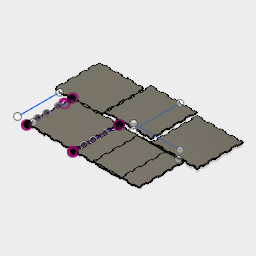
hezi2 v0 (Autodesk Fusion 360 design; units mm, degrees)
Autodesk Fusion 360 part; units mm, degrees
sketch "草图1" plane through (0, 0, 0) normal (0, 1, 0) x (1, 0, 0)
  line L0 (-50, 0) -> (30, 0)
  line L1 (30, 0) -> (30, -80)
  line L2 (30, -80) -> (-50, -80)
  line L3 (-50, -80) -> (-50, 0)
  line L4 (30, -10) -> (28, -10)
  line L5 (28, -10) -> (30, -10)
  line L6 (30, -10) -> (30, -20)
  line L7 (30, -20) -> (28, -20)
  line L8 (28, -20) -> (28, -10)
  line L9 (28, -30.1419) -> (30, -30.1419)
  line L10 (30, -30.1419) -> (30, -40)
  line L11 (30, -40) -> (28, -40)
  line L12 (28, -40) -> (28, -30.1419)
  line L13 (28, -49.9122) -> (30, -49.9122)
  line L14 (30, -49.9122) -> (30, -60)
  line L15 (30, -60) -> (28, -60)
  line L16 (28, -60) -> (28, -49.9122)
  line L17 (28, -70.124) -> (30, -70.124)
  line L18 (30, -70.124) -> (30, -80)
  line L19 (30, -80) -> (28, -80)
  line L20 (-50, -10) -> (-48, -10)
  line L21 (-48, -10) -> (-48, -19.9095)
  line L22 (-48, -19.9095) -> (-50, -19.9095)
  line L23 (-50, -19.9095) -> (-50, -10)
  line L24 (-48, -30.0089) -> (-50, -30.0089)
  line L25 (-50, -30.0089) -> (-50, -40)
  line L26 (-50, -40) -> (-48, -40)
  line L27 (-48, -40) -> (-48, -30.0089)
  line L28 (-48, -50.2335) -> (-50, -50.2335)
  line L29 (-50, -50.2335) -> (-50, -60)
  line L30 (-50, -60) -> (-48, -60)
  line L31 (-48, -60) -> (-48, -50.2335)
  line L32 (-50, -70.0828) -> (-50, -80)
  line L33 (-50, -80) -> (-48, -80)
  line L34 (-48, -70.0522) -> (-50, -70.0522)
  line L35 (-50, -70.0522) -> (-50, -75.0522)
  line L36 (-50, -75.0522) -> (-48, -75.0522)
  line L37 (-48, -75.0522) -> (-48, -70.0522)
  line L38 (28, -70.124) -> (30, -70.124)
  line L39 (30, -70.124) -> (30, -75.062)
  line L40 (30, -75.062) -> (28, -75.062)
  line L41 (28, -75.062) -> (28, -70.124)
  line L42 (-30, -80) -> (-19.728, -80)
  line L43 (-19.728, -80) -> (-19.728, -78)
  line L44 (-19.728, -78) -> (-30, -78)
  line L45 (-30, -78) -> (-30, -80)
  line L46 (-9.7551, -78) -> (0, -78)
  line L47 (0, -78) -> (0, -80)
  line L48 (0, -80) -> (-9.7551, -80)
  line L49 (-9.7551, -80) -> (-9.7551, -78)
  line L50 (-40.3031, -78) -> (-45.3133, -78)
  line L51 (-45.3133, -78) -> (-45.3133, -80)
  line L52 (-45.3133, -80) -> (-40.3031, -80)
  line L53 (-40.3031, -80) -> (-40.3031, -78)
  line L54 (-45.3133, 0) -> (-40.3031, 0)
  line L55 (-40.3031, 0) -> (-40.3031, -2)
  line L56 (-40.3031, -2) -> (-45.3133, -2)
  line L57 (-45.3133, -2) -> (-45.3133, 0)
  line L58 (-29.7585, -2) -> (-20, -2)
  line L59 (-20, -2) -> (-20, 0)
  line L60 (-20, 0) -> (-29.7585, 0)
  line L61 (-29.7585, 0) -> (-29.7585, -2)
  line L62 (-10, -2) -> (0, -2)
  line L63 (0, -2) -> (0, 0)
  line L64 (0, 0) -> (-10, 0)
  line L65 (-10, 0) -> (-10, -2)
  line L66 (10.2052, -2) -> (20, -2)
  line L67 (20, -2) -> (20, 0)
  line L68 (20, 0) -> (10.2052, 0)
  line L69 (10.2052, 0) -> (10.2052, -2)
  line L70 (10.3405, -78) -> (20, -78)
  line L71 (20, -78) -> (20, -80)
  line L72 (20, -80) -> (10.3405, -80)
  line L73 (10.3405, -80) -> (10.3405, -78)
  dimension "d1" = 80
  dimension "d2" = 80
  dimension "d3" = 2
  dimension "d4" = 2
  dimension "d5" = 5
  dimension "d6" = 2
  dimension "d7" = 2
  dimension "d8" = 2
  measures "d1" distance of L0.start L2.end
  measures "d2" distance of L0.start L0.end
  measures "d3" distance of L4.start L4.end
  measures "d4" distance of L20.start L20.end
  measures "d5" distance of L34.start L36.end
  measures "d6" distance of L17.start L17.end
  measures "d7" distance of L42.start L44.end
  measures "d8" distance of L54.start L56.end
extrude "拉伸1" add sketch "草图1" along normal blind 2 contours L0 L1 L2 L3 L4 L5 L7 L8 L9 L11 L12 L13 L15 L16 L17 L18 L19 L20 L21 L22 L24 L26 L27 L28 L30 L31 L32 L33 L34 L36 L37 L38 L40 L41 L43 L44 L45 L46 L47 L49 L50 L51 L53 L55 L56 L57 L58 L59 L61 L62 L63 L65 L66 L67 L69 L70 L71 L73 makes body 1
box "长方体基本要素1" add length 80 width 80 height 2 placed x (0, 0, 1) y (1, 0, 0) z (0, 1, 0) at (50, 0, 0) separate body makes body 2
sketch "草图3" plane through (0, 2, 0) normal (0, 1, 0) x (-1, 0, 0)
  line L0 (-50, 80) -> (-130, 80)
  line L1 (-130, 80) -> (-130, 0)
  line L2 (-130, 0) -> (-50, 0)
  line L3 (-50, 0) -> (-50, 80)
  line L4 (-50, 0) -> (-52, 0)
  line L5 (-52, 0) -> (-52, 9.9337)
  line L6 (-52, 9.9337) -> (-50, 9.9337)
  line L7 (-50, 9.9337) -> (-50, 0)
  line L8 (-52, 20.0066) -> (-50, 20.0066)
  line L9 (-50, 20.0066) -> (-50, 30)
  line L10 (-50, 30) -> (-52, 30)
  line L11 (-52, 30) -> (-52, 20.0066)
  line L12 (-52, 39.9379) -> (-50, 39.9379)
  line L13 (-50, 39.9379) -> (-50, 50)
  line L14 (-50, 50) -> (-52, 50)
  line L15 (-52, 50) -> (-52, 39.9379)
  line L16 (-52, 59.8692) -> (-50, 59.8692)
  line L17 (-50, 59.8692) -> (-50, 70)
  line L18 (-50, 70) -> (-52, 70)
  line L19 (-52, 70) -> (-52, 59.8692)
  line L20 (-52, 75.0856) -> (-50, 75.0856)
  line L21 (-50, 75.0856) -> (-50, 80)
  line L22 (-50, 80) -> (-52, 80)
  line L23 (-52, 80) -> (-52, 75.0856)
  line L24 (-130, 0) -> (-128, 0)
  line L25 (-128, 0) -> (-128, 9.9337)
  line L26 (-128, 9.9337) -> (-130, 9.9337)
  line L27 (-130, 9.9337) -> (-130, 0)
  line L28 (-128, 20.2209) -> (-130, 20.2209)
  line L29 (-130, 20.2209) -> (-130, 30)
  line L30 (-130, 30) -> (-128, 30)
  line L31 (-128, 30) -> (-128, 20.2209)
  line L32 (-128, 39.9379) -> (-130, 39.9379)
  line L33 (-130, 39.9379) -> (-130, 50)
  line L34 (-130, 50) -> (-128, 50)
  line L35 (-128, 50) -> (-128, 39.9379)
  line L36 (-128, 59.8692) -> (-130, 59.8692)
  line L37 (-130, 59.8692) -> (-130, 70)
  line L38 (-130, 70) -> (-128, 70)
  line L39 (-128, 70) -> (-128, 59.8692)
  line L40 (-128, 75.0856) -> (-130, 75.0856)
  line L41 (-130, 75.0856) -> (-130, 80)
  line L42 (-130, 80) -> (-128, 80)
  line L43 (-128, 80) -> (-128, 75.0856)
  line L44 (-55, 0) -> (-64.9634, 0)
  line L45 (-64.9634, 0) -> (-64.9634, 2)
  line L46 (-64.9634, 2) -> (-55, 2)
  line L47 (-55, 2) -> (-55, 0)
  line L48 (-75.0362, 2) -> (-85, 2)
  line L49 (-85, 2) -> (-85, 0)
  line L50 (-85, 0) -> (-75.0362, 0)
  line L51 (-75.0362, 0) -> (-75.0362, 2)
  line L52 (-94.9675, 2) -> (-105, 2)
  line L53 (-105, 2) -> (-105, 0)
  line L54 (-105, 0) -> (-94.9675, 0)
  line L55 (-94.9675, 0) -> (-94.9675, 2)
  line L56 (-109.9696, 2) -> (-120, 2)
  line L57 (-120, 2) -> (-120, 0)
  line L58 (-120, 0) -> (-109.9696, 0)
  line L59 (-109.9696, 0) -> (-109.9696, 2)
  line L60 (-55, 80) -> (-64.9634, 80)
  line L61 (-64.9634, 80) -> (-64.9634, 78)
  line L62 (-64.9634, 78) -> (-55, 78)
  line L63 (-55, 78) -> (-55, 80)
  line L64 (-75.2505, 78) -> (-85, 78)
  line L65 (-85, 78) -> (-85, 80)
  line L66 (-85, 80) -> (-75.2505, 80)
  line L67 (-75.2505, 80) -> (-75.2505, 78)
  line L68 (-94.9675, 78) -> (-105, 78)
  line L69 (-105, 78) -> (-105, 80)
  line L70 (-105, 80) -> (-94.9675, 80)
  line L71 (-94.9675, 80) -> (-94.9675, 78)
  line L72 (-109.9696, 78) -> (-120, 78)
  line L73 (-120, 78) -> (-120, 80)
  line L74 (-120, 80) -> (-109.9696, 80)
  line L75 (-109.9696, 80) -> (-109.9696, 78)
  dimension "d16" = 2
  measures "d16" distance of L2.end L4.end
extrude "拉伸2" add sketch "草图3" along normal blind 2 contours L0 L1 L2 L3 L5 L6 L8 L10 L11 L12 L14 L15 L16 L18 L19 L20 L23 L25 L26 L28 L30 L31 L32 L34 L35 L36 L38 L39 L40 L43 L45 L46 L47 L48 L49 L51 L52 L53 L55 L56 L57 L59 L61 L62 L63 L64 L65 L67 L68 L69 L71 L72 L73 L75 bodies 2
sketch "草图4" plane through (0, 0, 0) normal (0, 0, -1) x (-1, 0, 0)
  line L0 (-130, 2) -> (-130, 0)
  line L1 (-130, 0) -> (-50, 0)
  line L2 (-50, 0) -> (-50, 2)
  line L3 (-50, 2) -> (-52, 2)
  line L4 (-52, 2) -> (-52, 4)
  line L5 (-52, 4) -> (-55, 4)
  line L6 (-55, 4) -> (-55, 2)
  line L7 (-55, 2) -> (-64.9634, 2)
  line L8 (-64.9634, 2) -> (-64.9634, 4)
  line L9 (-64.9634, 4) -> (-75.0362, 4)
  line L10 (-75.0362, 4) -> (-75.0362, 2)
  line L11 (-75.0362, 2) -> (-85, 2)
  line L12 (-85, 2) -> (-85, 4)
  line L13 (-85, 4) -> (-94.9675, 4)
  line L14 (-94.9675, 4) -> (-94.9675, 2)
  line L15 (-94.9675, 2) -> (-105, 2)
  line L16 (-105, 2) -> (-105, 4)
  line L17 (-105, 4) -> (-109.9696, 4)
  line L18 (-109.9696, 4) -> (-109.9696, 2)
  line L19 (-109.9696, 2) -> (-120, 2)
  line L20 (-120, 2) -> (-120, 4)
  line L21 (-120, 4) -> (-128, 4)
  line L22 (-128, 4) -> (-128, 2)
  line L23 (-128, 2) -> (-130, 2)
  line L24 (-130, 2) -> (-50, 2)
  line L25 (-50, 2) -> (-50, 0)
  line L26 (-50, 0) -> (-130, 0)
  line L27 (-130, 0) -> (-130, 2)
extrude "拉伸3" cut sketch "草图4" against normal blind 80 contours L0 L1 L2 L3 L7 L11 L15 L19 L23 L24 L25 L26 L27 bodies 2
move_body "移动1" bodies 2 to x (1, 0, 0) y (0, 1, 0) z (0, 0, 1) at (0, -2, 0)
sketch "草图5" plane through (0, 2, 0) normal (0, 1, 0) x (-1, 0, 0)
  line L0 (9.7551, 80) -> (9.7551, 78)
  line L1 (9.7551, 78) -> (0, 78)
  line L2 (0, 78) -> (0, 80)
  line L3 (0, 80) -> (-10.3405, 80)
  line L4 (-10.3405, 80) -> (-10.3405, 78)
  line L5 (-10.3405, 78) -> (-20, 78)
  line L6 (-20, 78) -> (-20, 80)
  line L7 (-20, 80) -> (-30, 80)
  line L8 (-30, 80) -> (-30, 75.062)
  line L9 (-30, 75.062) -> (-28, 75.062)
  line L10 (-28, 75.062) -> (-28, 70.124)
  line L11 (-28, 70.124) -> (-30, 70.124)
  line L12 (-30, 70.124) -> (-30, 60)
  line L13 (-30, 60) -> (-28, 60)
  line L14 (-28, 60) -> (-28, 49.9122)
  line L15 (-28, 49.9122) -> (-30, 49.9122)
  line L16 (-30, 49.9122) -> (-30, 40)
  line L17 (-30, 40) -> (-28, 40)
  line L18 (-28, 40) -> (-28, 30.1419)
  line L19 (-28, 30.1419) -> (-30, 30.1419)
  line L20 (-30, 30.1419) -> (-30, 20)
  line L21 (-30, 20) -> (-28, 20)
  line L22 (-28, 20) -> (-28, 10)
  line L23 (-28, 10) -> (-30, 10)
  line L24 (-30, 10) -> (-30, 0)
  line L25 (-30, 0) -> (-20, 0)
  line L26 (-20, 0) -> (-20, 2)
  line L27 (-20, 2) -> (-10.2052, 2)
  line L28 (-10.2052, 2) -> (-10.2052, 0)
  line L29 (-10.2052, 0) -> (0, 0)
  line L30 (0, 0) -> (0, 2)
  line L31 (0, 2) -> (10, 2)
  line L32 (10, 2) -> (10, 0)
  line L33 (10, 0) -> (20, 0)
  line L34 (20, 0) -> (20, 2)
  line L35 (20, 2) -> (29.7585, 2)
  line L36 (29.7585, 2) -> (29.7585, 0)
  line L37 (29.7585, 0) -> (40.3031, 0)
  line L38 (40.3031, 0) -> (40.3031, 2)
  line L39 (40.3031, 2) -> (45.3133, 2)
  line L40 (45.3133, 2) -> (45.3133, 0)
  line L41 (45.3133, 0) -> (50, 0)
  line L42 (50, 0) -> (50, 10)
  line L43 (50, 10) -> (48, 10)
  line L44 (48, 10) -> (48, 19.9095)
  line L45 (48, 19.9095) -> (50, 19.9095)
  line L46 (50, 19.9095) -> (50, 30.0089)
  line L47 (50, 30.0089) -> (48, 30.0089)
  line L48 (48, 30.0089) -> (48, 40)
  line L49 (48, 40) -> (50, 40)
  line L50 (50, 40) -> (50, 50.2335)
  line L51 (50, 50.2335) -> (48, 50.2335)
  line L52 (48, 50.2335) -> (48, 60)
  line L53 (48, 60) -> (50, 60)
  line L54 (50, 60) -> (50, 70.0522)
  line L55 (50, 70.0522) -> (48, 70.0522)
  line L56 (48, 70.0522) -> (48, 75.0522)
  line L57 (48, 75.0522) -> (50, 75.0522)
  line L58 (50, 75.0522) -> (50, 80)
  line L59 (50, 80) -> (45.3133, 80)
  line L60 (45.3133, 80) -> (45.3133, 78)
  line L61 (45.3133, 78) -> (40.3031, 78)
  line L62 (40.3031, 78) -> (40.3031, 80)
  line L63 (40.3031, 80) -> (30, 80)
  line L64 (30, 80) -> (30, 78)
  line L65 (30, 78) -> (19.728, 78)
  line L66 (19.728, 78) -> (19.728, 80)
  line L67 (19.728, 80) -> (9.7551, 80)
  line L68 (50, 85) -> (-30, 85)
  line L69 (-30, 85) -> (-30, 165)
  line L70 (-30, 165) -> (50, 165)
  line L71 (50, 165) -> (50, 85)
  line L72 (50, 85) -> (45.3133, 85)
  line L73 (45.3133, 85) -> (45.3133, 87)
  line L74 (45.3133, 87) -> (50, 87)
  line L75 (50, 87) -> (50, 85)
  line L76 (40.0206, 87) -> (30.0852, 87)
  line L77 (30.0852, 87) -> (30.0852, 85)
  line L78 (30.0852, 85) -> (40.0206, 85)
  line L79 (40.0206, 85) -> (40.0206, 87)
  line L80 (19.9188, 87) -> (10, 87)
  line L81 (10, 87) -> (10, 85)
  line L82 (10, 85) -> (19.9188, 85)
  line L83 (19.9188, 85) -> (19.9188, 87)
  line L84 (0.048, 87) -> (-10.5806, 87)
  line L85 (-10.5806, 87) -> (-10.5806, 85)
  line L86 (-10.5806, 85) -> (0.048, 85)
  line L87 (0.048, 85) -> (0.048, 87)
  line L88 (-20.2849, 87) -> (-30, 87)
  line L89 (-30, 87) -> (-30, 85)
  line L90 (-30, 85) -> (-20.2849, 85)
  line L91 (-20.2849, 85) -> (-20.2849, 87)
  line L92 (45.3133, 165) -> (50, 165)
  line L93 (50, 165) -> (50, 163)
  line L94 (50, 163) -> (45.3133, 163)
  line L95 (45.3133, 163) -> (45.3133, 165)
  line L96 (40.0206, 163) -> (29.8542, 163)
  line L97 (29.8542, 163) -> (29.8542, 165)
  line L98 (29.8542, 165) -> (40.0206, 165)
  line L99 (40.0206, 165) -> (40.0206, 163)
  line L100 (19.9188, 163) -> (10, 163)
  line L101 (10, 163) -> (10, 165)
  line L102 (10, 165) -> (19.9188, 165)
  line L103 (19.9188, 165) -> (19.9188, 163)
  line L104 (-0.1831, 163) -> (-10.1185, 163)
  line L105 (-10.1185, 163) -> (-10.1185, 165)
  line L106 (-10.1185, 165) -> (-0.1831, 165)
  line L107 (-0.1831, 165) -> (-0.1831, 163)
  line L108 (-20.0539, 163) -> (-30, 163)
  line L109 (-30, 163) -> (-30, 165)
  line L110 (-30, 165) -> (-20.0539, 165)
  line L111 (-20.0539, 165) -> (-20.0539, 163)
  dimension "d21" = 80
  dimension "d22" = 80
  dimension "d23" = 2
  dimension "d24" = 2
  measures "d21" distance of L68.start L70.end
  measures "d22" distance of L68.start L68.end
  measures "d23" distance of L68.start L74.end
  measures "d24" distance of L92.start L94.end
move_body "移动2" bodies 2 to x (1, 0, 0) y (0, 1, 0) z (0, 0, 1) at (0, 0, 85)
sketch "草图6" plane through (0, 0, 0) normal (0, 1, 0) x (1, 0, 0)
  line L0 (30, -85) -> (30, -165)
  line L1 (30, -85) -> (132.5104, -85)
  point P0 (30, -85)
move_face "MoveFace1" to x (0, 0, 1) y (0, 1, 0) z (-1, 0, 0) at (174.9428, 0, 36.9961) 1 faces at (91.6558, 2, 137.6253) on bodies 2
move_body "移动3" bodies 2 to x (0, 0, 1) y (0, 1, 0) z (-1, 0, 0) at (197.9117, 0, 33.4081)
move_body "移动4" bodies 2 to x (1, 0, 0) y (0, 1, 0) z (0, 0, 1) at (0, 0, 2)
sketch "草图7" plane through (0, 0, 0) normal (0, 1, 0) x (1, 0, 0)
  line L0 (30, -87) -> (28, -87)
  line L1 (28, -87) -> (28, -90.3428)
  line L2 (28, -90.3428) -> (30, -90.3428)
  line L3 (30, -90.3428) -> (30, -87)
  line L4 (28, -100.0471) -> (30, -100.0471)
  line L5 (30, -100.0471) -> (30, -110)
  line L6 (30, -110) -> (28, -110)
  line L7 (28, -110) -> (28, -100.0471)
  line L8 (30, -85) -> (30, -165)
  line L9 (28, -120.38) -> (30, -120.38)
  line L10 (30, -120.38) -> (30, -130)
  line L11 (30, -130) -> (28, -130)
  line L12 (28, -130) -> (28, -120.38)
  line L13 (28, -140.2508) -> (30, -140.2508)
  line L14 (30, -140.2508) -> (30, -145.334)
  line L15 (30, -145.334) -> (28, -145.334)
  line L16 (28, -145.334) -> (28, -140.2508)
  line L17 (28, -155.5004) -> (30, -155.5004)
  line L18 (30, -155.5004) -> (30, -163)
  line L19 (30, -163) -> (28, -163)
  line L20 (28, -163) -> (28, -155.5004)
  line L21 (-50, -87) -> (-48, -87)
  line L22 (-48, -87) -> (-48, -90.3428)
  line L23 (-48, -90.3428) -> (-50, -90.3428)
  line L24 (-50, -90.3428) -> (-50, -87)
  line L25 (-48, -100.2781) -> (-50, -100.2781)
  line L26 (-50, -100.2781) -> (-50, -110)
  line L27 (-50, -110) -> (-48, -110)
  line L28 (-48, -110) -> (-48, -100.2781)
  line L29 (-50, -165) -> (-50, -85)
  line L30 (-48, -119.9179) -> (-50, -119.9179)
  line L31 (-50, -119.9179) -> (-50, -130)
  line L32 (-50, -130) -> (-48, -130)
  line L33 (-48, -130) -> (-48, -119.9179)
  line L34 (-48, -140.2508) -> (-50, -140.2508)
  line L35 (-50, -140.2508) -> (-50, -145.334)
  line L36 (-50, -145.334) -> (-48, -145.334)
  line L37 (-48, -145.334) -> (-48, -140.2508)
  line L38 (-50, -163) -> (-48, -163)
  line L39 (-48, -155.5004) -> (-50, -155.5004)
  line L40 (-50, -155.5004) -> (-50, -163)
  line L41 (-50, -155.5004) -> (-48, -155.5004)
  line L42 (-48, -155.5004) -> (-48, -163)
  line L43 (-48, -163) -> (-50, -163)
  line L44 (-50, -163) -> (-50, -155.5004)
  point P0 (30, -87)
  point P1 (30, -163)
  point P2 (-50, -87)
  point P3 (-50, -163)
  dimension "d25" = 2
  dimension "d26" = 2
  measures "d25" distance of P0 L0.end
  measures "d26" distance of P3 L38.end
extrude "拉伸4" add sketch "草图5" along normal blind 2 separate body contours L68 L69 L70 L71 L73 L74 L76 L77 L79 L80 L81 L83 L84 L85 L87 L88 L91 L94 L95 L96 L97 L99 L100 L101 L103 L104 L105 L107 L108 L111 makes body 3
sketch "草图8" plane through (0, 4, 0) normal (0, 1, 0) x (-1, 0, 0)
  line L0 (-0.1831, 165) -> (-0.1831, 163)
  line L1 (-0.1831, 163) -> (-10.1185, 163)
  line L2 (-10.1185, 163) -> (-10.1185, 165)
  line L3 (-10.1185, 165) -> (-20.0539, 165)
  line L4 (-20.0539, 165) -> (-20.0539, 163)
  line L5 (-20.0539, 163) -> (-30, 163)
  line L6 (-30, 163) -> (-30, 87)
  line L7 (-30, 87) -> (-20.2849, 87)
  line L8 (-20.2849, 87) -> (-20.2849, 85)
  line L9 (-20.2849, 85) -> (-10.5806, 85)
  line L10 (-10.5806, 85) -> (-10.5806, 87)
  line L11 (-10.5806, 87) -> (0.048, 87)
  line L12 (0.048, 87) -> (0.048, 85)
  line L13 (0.048, 85) -> (10, 85)
  line L14 (10, 85) -> (10, 87)
  line L15 (10, 87) -> (19.9188, 87)
  line L16 (19.9188, 87) -> (19.9188, 85)
  line L17 (19.9188, 85) -> (30.0852, 85)
  line L18 (30.0852, 85) -> (30.0852, 87)
  line L19 (30.0852, 87) -> (40.0206, 87)
  line L20 (40.0206, 87) -> (40.0206, 85)
  line L21 (40.0206, 85) -> (45.3133, 85)
  line L22 (45.3133, 85) -> (45.3133, 87)
  line L23 (45.3133, 87) -> (50, 87)
  line L24 (50, 87) -> (50, 163)
  line L25 (50, 163) -> (45.3133, 163)
  line L26 (45.3133, 163) -> (45.3133, 165)
  line L27 (45.3133, 165) -> (40.0206, 165)
  line L28 (40.0206, 165) -> (40.0206, 163)
  line L29 (40.0206, 163) -> (29.8542, 163)
  line L30 (29.8542, 163) -> (29.8542, 165)
  line L31 (29.8542, 165) -> (19.9188, 165)
  line L32 (19.9188, 165) -> (19.9188, 163)
  line L33 (19.9188, 163) -> (10, 163)
  line L34 (10, 163) -> (10, 165)
  line L35 (10, 165) -> (-0.1831, 165)
  line L36 (-28, 87) -> (-30, 87)
  line L37 (-30, 87) -> (-30, 90.3428)
  line L38 (-30, 90.3428) -> (-28, 90.3428)
  line L39 (-28, 90.3428) -> (-28, 87)
  line L40 (-28, 100.0471) -> (-30, 100.0471)
  line L41 (-30, 100.0471) -> (-30, 110)
  line L42 (-30, 110) -> (-28, 110)
  line L43 (-28, 110) -> (-28, 100.0471)
  line L44 (-28, 120.38) -> (-30, 120.38)
  line L45 (-30, 120.38) -> (-30, 130)
  line L46 (-30, 130) -> (-28, 130)
  line L47 (-28, 130) -> (-28, 120.38)
  line L48 (-28, 140.2508) -> (-30, 140.2508)
  line L49 (-30, 140.2508) -> (-30, 145.334)
  line L50 (-30, 145.334) -> (-28, 145.334)
  line L51 (-28, 145.334) -> (-28, 140.2508)
  line L52 (-28, 155.5004) -> (-30, 155.5004)
  line L53 (-30, 155.5004) -> (-30, 163)
  line L54 (-30, 163) -> (-28, 163)
  line L55 (-28, 163) -> (-28, 155.5004)
  line L56 (50, 87) -> (48, 87)
  line L57 (48, 87) -> (48, 90.3428)
  line L58 (48, 90.3428) -> (50, 90.3428)
  line L59 (50, 90.3428) -> (50, 87)
  line L60 (50, 100.2781) -> (48, 100.2781)
  line L61 (48, 100.2781) -> (48, 110)
  line L62 (48, 110) -> (50, 110)
  line L63 (50, 110) -> (50, 100.2781)
  line L64 (50, 119.9179) -> (48, 119.9179)
  line L65 (48, 119.9179) -> (48, 130)
  line L66 (48, 130) -> (50, 130)
  line L67 (50, 130) -> (50, 119.9179)
  line L68 (50, 140.2508) -> (48, 140.2508)
  line L69 (48, 140.2508) -> (48, 145.334)
  line L70 (48, 145.334) -> (50, 145.334)
  line L71 (50, 145.334) -> (50, 140.2508)
  line L72 (50, 155.5004) -> (48, 155.5004)
  line L73 (48, 155.5004) -> (48, 163)
  line L74 (48, 163) -> (50, 163)
  line L75 (50, 163) -> (50, 155.5004)
  point P0 (-28, 87)
  point P1 (-30, 90.3428)
  point P2 (-28, 100.0471)
  point P3 (-30, 110)
  point P4 (-28, 120.38)
  point P5 (-30, 130)
  point P6 (-28, 140.2508)
  point P7 (-30, 145.334)
  point P8 (-28, 155.5004)
  point P9 (48, 90.3428)
  point P10 (50, 100.2781)
  point P11 (48, 110)
  point P12 (50, 119.9179)
  point P13 (48, 130)
  point P14 (50, 140.2508)
  point P15 (48, 145.334)
  point P16 (50, 155.5004)
  point P17 (48, 163)
extrude "拉伸5" add sketch "草图8" along normal blind 2 contours L0 L1 L2 L3 L4 L5 L6 L7 L8 L9 L10 L11 L12 L13 L14 L15 L16 L17 L18 L19 L20 L21 L22 L23 L24 L25 L26 L27 L28 L29 L30 L31 L32 L33 L34 L35 L38 L39 L40 L42 L43 L44 L46 L47 L48 L50 L51 L52 L55 L57 L58 L60 L61 L62 L64 L65 L66 L68 L69 L70 L72 L73 bodies 3
sketch "草图9" plane through (-50, 0, 0) normal (-1, 0, 0) x (0, 0, 1)
  line L0 (87, 2) -> (163, 2)
  line L1 (163, 2) -> (163, 4)
  line L2 (163, 4) -> (155.5004, 4)
  line L3 (155.5004, 4) -> (155.5004, 6)
  line L4 (155.5004, 6) -> (145.334, 6)
  line L5 (145.334, 6) -> (145.334, 4)
  line L6 (145.334, 4) -> (140.2508, 4)
  line L7 (140.2508, 4) -> (140.2508, 6)
  line L8 (140.2508, 6) -> (130, 6)
  line L9 (130, 6) -> (130, 4)
  line L10 (130, 4) -> (119.9179, 4)
  line L11 (119.9179, 4) -> (119.9179, 6)
  line L12 (119.9179, 6) -> (110, 6)
  line L13 (110, 6) -> (110, 4)
  line L14 (110, 4) -> (100.2781, 4)
  line L15 (100.2781, 4) -> (100.2781, 6)
  line L16 (100.2781, 6) -> (90.3428, 6)
  line L17 (90.3428, 6) -> (90.3428, 4)
  line L18 (90.3428, 4) -> (87, 4)
  line L19 (87, 4) -> (87, 2)
  line L20 (87, 2) -> (163, 2)
  line L21 (163, 2) -> (163, 4)
  line L22 (163, 4) -> (87, 4)
  line L23 (87, 4) -> (87, 2)
extrude "拉伸6" cut sketch "草图9" against normal blind 80 contours L0 L1 L2 L6 L10 L14 L18 L19 L20 L21 L22 L23 bodies 3
sketch "草图10" plane through (0, 0, 165) normal (0, 0, 1) x (1, 0, 0)
  line L0 (-45.3133, 2) -> (-40.0206, 2)
  line L1 (-40.0206, 2) -> (-40.0206, 6)
  line L2 (-40.0206, 6) -> (-45.3133, 6)
  line L3 (-45.3133, 6) -> (-45.3133, 2)
  line L4 (-45.3133, 2) -> (-40.0206, 2)
  line L5 (-40.0206, 2) -> (-40.0206, 4)
  line L6 (-40.0206, 4) -> (-45.3133, 4)
  line L7 (-45.3133, 4) -> (-45.3133, 2)
  line L8 (-29.8542, 2) -> (-19.9463, 2)
  line L9 (-19.9463, 2) -> (-19.9463, 4)
  line L10 (-19.9463, 4) -> (-29.8542, 4)
  line L11 (-29.8542, 4) -> (-29.8542, 2)
  line L12 (-30.0852, 4) -> (-19.9188, 4)
  line L13 (-10, 2) -> (0.1831, 2)
  line L14 (0.1831, 2) -> (0.1831, 4)
  line L15 (0.1831, 4) -> (-10, 4)
  line L16 (-10, 4) -> (-10, 2)
  line L17 (10.1185, 2) -> (20.0539, 2)
  line L18 (20.0539, 2) -> (20.0539, 4)
  line L19 (20.0539, 4) -> (10.1185, 4)
  line L20 (10.1185, 4) -> (10.1185, 2)
  line L21 (20.0539, 2) -> (20.0539, 6)
  point P0 (-40.0206, 4)
  point P1 (-29.8542, 2)
  point P2 (-10, 2)
  point P3 (0.1831, 4)
  point P4 (10.1185, 2)
extrude "拉伸7" cut sketch "草图10" against normal blind 65 contours L0 L1 L3 L4 L5 L6 L7 | L8 L9 L10 L11 L12 | L13 L14 L15 L16 | L17 L18 L19 L20 L21 bodies 3
sketch "草图11" plane through (0, 0, 85) normal (0, 0, -1) x (-1, 0, 0)
  line L0 (-20.2849, 2) -> (-10.5806, 2)
  line L1 (-10.5806, 2) -> (-10.5806, 6)
  line L2 (-10.5806, 6) -> (-20.2849, 6)
  line L3 (-20.2849, 6) -> (-20.2849, 2)
  line L4 (-20.2849, 2) -> (-10.5806, 2)
  line L5 (-10.5806, 2) -> (-10.5806, 4)
  line L6 (-10.5806, 4) -> (-20.2849, 4)
  line L7 (-20.2849, 4) -> (-20.2849, 2)
  line L8 (0, 2) -> (10, 2)
  line L9 (10, 2) -> (10, 4)
  line L10 (10, 4) -> (0, 4)
  line L11 (0, 4) -> (0, 2)
  line L12 (20, 2) -> (30.0216, 2)
  line L13 (30.0216, 2) -> (30.0216, 4)
  line L14 (30.0216, 4) -> (20, 4)
  line L15 (20, 4) -> (20, 2)
  line L16 (30.0852, 4) -> (19.9188, 4)
  line L17 (40.3031, 2) -> (44.994, 2)
  line L18 (44.994, 2) -> (44.994, 4)
  line L19 (44.994, 4) -> (40.3031, 4)
  line L20 (40.3031, 4) -> (40.3031, 2)
  line L21 (45.3133, 4) -> (40.0206, 4)
  point P0 (-10.5806, 4)
  point P1 (0, 2)
  point P2 (10, 4)
  point P3 (20, 2)
  point P4 (40.3031, 2)
extrude "拉伸8" cut sketch "草图11" against normal blind 35 contours L0 L1 L3 L4 L5 L6 L7 | L8 L9 L10 L11 | L12 L13 L14 L15 L16 | L17 L18 L19 L20 L21 bodies 3
move_body "移动5" bodies 3 to x (1, 0, 0) y (0, 1, 0) z (0, 0, 1) at (0, -4, 0)
sketch "草图12" plane through (0, 0, 0) normal (0, 0, 1) x (1, 0, 0)
sketch "草图13" plane through (0, 0, 0) normal (0, 1, 0) x (1, 0, 0)
  line L0 (50, 0) -> (50, -80)
  line L1 (40, -70) -> (120, -70)
  line L2 (-48, -100.2781) -> (-50, -100.2781)
  line L3 (-70.39, -87.4081) -> (-70.39, -160)
mirror "镜像1" about plane through (0, 0, 0) normal (0, 0, 1) of bodies 2 makes body 4
mirror "镜像2" about plane through (0, 0, 0) normal (1, 0, 0) of bodies 1 makes body 5
mirror "镜像3" about plane through (0, 0, 0) normal (0, 0, 1) of bodies 3 makes body 6
move_body "移动6" bodies 5 to x (1, 0, 0) y (0, 1, 0) z (0, 0, 1) at (30, 0, 0)
move_body "移动7" bodies 4 to x (1, 0, 0) y (0, 1, 0) z (0, 0, 1) at (30, 0, 250)
move_body "移动8" bodies 6 to x (1, 0, 0) y (0, 1, 0) z (0, 0, 1) at (-40, 0, 250)
move_body "移动9" bodies 1 to x (1, 0, 0) y (0, 1, 0) z (0, 0, 1) at (0, 78, 0)
move_body "移动10" bodies 1 to x (-1, 0, 0) y (0, -1, 0) z (0, 0, 1) at (28.5692, 160, 0)
move_body "移动11" bodies 6 to x (-1, 0, 0) y (0, 0, 1) z (0, 1, 0) at (-10.5532, -84.8776, -0.1224)
move_body "对齐1" bodies 1 to x (1, 0, 0) y (0, 1, 0) z (0, 0, 1) at (0, 0, -0.1224)
move_body "移动12" bodies 1 to x (1, 0, 0) y (0, 1, 0) z (0, 0, 1) at (47.724, -78.4456, -13.3943)
move_body "移动13" bodies 6 to x (1, 0, 0) y (0, 0, 1) z (0, -1, 0) at (-80, 1.2454, 8.5098)
move_body "移动14" bodies 1 to x (1, 0, 0) y (0, 1, 0) z (0, 0, 1) at (40, 0, 20)
